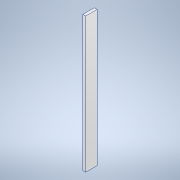
# Autodesk Inventor part: 14in-slide-pt_3
Saved by Autodesk Inventor 2020.1 (Build 241239000, 239)
## iProperties
Created: 2019-09-13
Part Number: 14in-slide-pt_3
Material: Aluminum 6061
Document SubType Name: Modeling
Designer: alpha
Density: 2.7 g/cm^3
Appearance: Aluminum - Flat
Author: alpha
Autodesk Inventor part; units mm, degrees
ref_plane "YZ Plane" through (0, 0, 0) normal (1, 0, 0) x (0, 1, 0)
ref_plane "XZ Plane" through (0, 0, 0) normal (0, 1, 0) x (-1, 0, 0)
ref_plane "XY Plane" through (0, 0, 0) normal (0, 0, 1) x (1, 0, 0)
sketch "Sketch1" plane through (0, 0, 0) normal (0, 1, 0) x (-1, 0, 0)
  line L0 (-3.175, -12.7) -> (3.175, -12.7)
  line L1 (3.175, -12.7) -> (3.175, 12.7)
  line L2 (3.175, 12.7) -> (-3.175, 12.7)
  line L3 (-3.175, 12.7) -> (-3.175, -12.7)
  line L4 (-3.175, -12.7) -> (3.175, 12.7) construction
  line L5 (3.175, -12.7) -> (-3.175, 12.7) construction
  point P0 (0, 0)
  dimension "d0" = 6.35
  dimension "d1" = 25.4
  constraints: 12 end point, 2 midpoint, 2 parallel, 1 horizontal, 1 perpendicular
  measures "d0" distance of L2.end L1.end
  measures "d1" distance of L1.end L0.end
extrude "Extrusion1" add sketch "Sketch1" along normal blind 304.8
body "Solid1"
